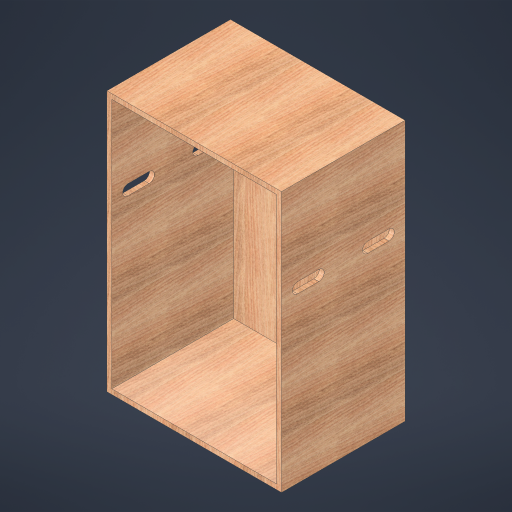
# Autodesk Inventor part: old battery cart
Saved by Autodesk Inventor 2023.4 (Build 274418000, 418)
## iProperties
Created: 2025-03-02
Part Number: old battery cart
Material: Wood (Birch)
Document SubType Name: Modeling
Designer: brand
Density: 0.55 g/cm^3
Appearance: Birch - Natural Polished
Author: brand
Autodesk Inventor part; units mm, degrees
ref_plane "YZ Plane" through (0, 0, 0) normal (1, 0, 0) x (0, 1, 0)
ref_plane "XZ Plane" through (0, 0, 0) normal (0, 1, 0) x (-1, 0, 0)
ref_plane "XY Plane" through (0, 0, 0) normal (0, 0, 1) x (1, 0, 0)
sketch "Sketch1" plane through (0, 0, 0) normal (0, 0, 1) x (1, 0, 0)
  line L0 (-292.1, -444.5) -> (292.1, -444.5)
  line L1 (292.1, -444.5) -> (292.1, 444.5)
  line L2 (292.1, 444.5) -> (-292.1, 444.5)
  line L3 (-292.1, 444.5) -> (-292.1, -444.5)
  line L4 (-292.1, -444.5) -> (292.1, 444.5) construction
  line L5 (292.1, -444.5) -> (-292.1, 444.5) construction
  line L6 (-309.626, 462.026) -> (309.626, 462.026)
  line L7 (309.626, 462.026) -> (309.626, -462.026)
  line L8 (309.626, -462.026) -> (-309.626, -462.026)
  line L9 (-309.626, -462.026) -> (-309.626, 462.026)
  point P0 (0, 0)
  dimension "d0" = 584.2
  dimension "d1" = 889
  dimension "d4" = 17.526
  constraints: 20 end point, 4 parallel, 2 midpoint, 2 perpendicular, 1 horizontal, 3 other
  measures "d0" distance of L2.end L1.end
  measures "d1" distance of L1.end L0.end
  measures "d4" distance between parallel lines of L2 L6
extrude "Extrusion1" add sketch "Sketch1" against normal blind 438.15 contours L3 L2 L1 L0 | L6 L7 L8 L9
extrude "Extrusion2" cut sketch "Sketch1" against normal blind 431.8 contours L3 L2 L1 L0
sketch "Sketch3" plane through (-309.626, -462.026, 0) normal (-1, 0, 0) x (0, 0, 1)
  line L0 (0, 0) -> (-438.15, 0) construction
  line L1 (-438.15, 0) -> (-438.15, 924.052) construction
  line L2 (-438.15, 924.052) -> (0, 924.052) construction
  line L3 (0, 924.052) -> (0, 0) construction
  line L4 (-38.1, 600.456) -> (-151.13, 600.456) construction
  line L5 (-56.896, 619.252) -> (-132.334, 619.252)
  line L6 (-132.334, 581.66) -> (-56.896, 581.66)
  arc A0 (-56.896, 581.66) -> (-56.896, 619.252) centre (-56.896, 600.456) ccw
  arc A1 (-132.334, 619.252) -> (-132.334, 581.66) centre (-132.334, 600.456) ccw
  line L7 (-287.02, 600.456) -> (-400.05, 600.456) construction
  line L8 (-305.816, 619.252) -> (-381.254, 619.252)
  line L9 (-381.254, 581.66) -> (-305.816, 581.66)
  arc A2 (-305.816, 581.66) -> (-305.816, 619.252) centre (-305.816, 600.456) ccw
  arc A3 (-381.254, 619.252) -> (-381.254, 581.66) centre (-381.254, 600.456) ccw
  point P0 (0, 462.026)
  point P1 (-94.615, 600.456)
  point P2 (-343.535, 600.456)
  point P3 (-38.1, 600.456)
  point P4 (-400.05, 600.456)
  dimension "d7" = 113.03
  dimension "d8" = 37.592
  dimension "d9" = 113.03
  dimension "d10" = 38.1
  dimension "d11" = 304.8
  dimension "d12" = 38.1
  constraints: 16 end point, 14 point on circle, 8 tangent, 6 point on line, 4 centre point, 2 horizontal alignment, 2 midpoint, 2 parallel, 1 horizontal
  measures "d7" distance of L4.start L4.end
  measures "d8" distance between parallel lines of L6 L5
  measures "d9" distance of L7.start L7.end
  measures "d10" distance from line of L3 point (-38.1, 600.456)
  measures "d11" distance between parallel lines of L2 L5
  measures "d12" distance from line of L1 point (-400.05, 600.456)
extrude "Extrusion3" cut sketch "Sketch3" against normal through all
equation "\"d9\" = d7"
body "Solid1"
